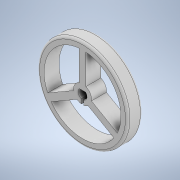
# Autodesk Inventor part: wheel35mmV1
Saved by Autodesk Inventor 2022.2 (Build 262287010, 287A)
## iProperties
Created: 2022-02-20
Part Number: wheel35mmV1
Material: Generic
Document SubType Name: Modeling
Designer: Nakai
Density: 1 g/cm^3
Appearance: Default
Author: Nakai
Autodesk Inventor part; units mm, degrees
ref_plane "YZ Plane" through (0, 0, 0) normal (1, 0, 0) x (0, 1, 0)
ref_plane "XZ Plane" through (0, 0, 0) normal (0, 1, 0) x (-1, 0, 0)
ref_plane "XY Plane" through (0, 0, 0) normal (0, 0, 1) x (1, 0, 0)
sketch "Sketch1" plane through (0, 0, 0) normal (0, 0, 1) x (1, 0, 0)
  circle A0 centre (0, 0) radius 20
  dimension "d0" = 40
  constraints: 1 centre point, 1 coincident
  measures "d0" diameter of A0
extrude "Extrusion1" add sketch "Sketch1" along normal blind 6.6
sketch "Sketch3" plane through (0, 0, 0) normal (0, 0, -1) x (-1, 0, 0)
  circle A0 centre (0, 0) radius 17
  line L0 (0, 17) -> (0, 0)
  line L1 (0, 0) -> (14.7224, -8.5)
  line L2 (0, 0) -> (-14.7224, -8.5)
  line L3 (0, 0) -> (17, 0) construction
  line L4 (1.5, 16.9337) -> (1.5, 0.866)
  line L5 (-1.5, 16.9337) -> (-1.5, 0.866)
  line L6 (-1.5, 0.866) -> (-15.415, -7.1678)
  line L7 (0, -1.7321) -> (-13.915, -9.7659)
  line L8 (1.5, 0.866) -> (15.415, -7.1678)
  line L9 (0, -1.7321) -> (13.915, -9.7659)
  dimension "d6" = 34
  dimension "d7" = 120
  dimension "d8" = 150
  dimension "d9" = 1.5
  dimension "d10" = 1.5
  dimension "d11" = 1.5
  dimension "d12" = 1.5
  dimension "d13" = 1.5
  dimension "d14" = 1.5
  constraints: 20 end point, 6 parallel, 1 coincident, 1 equal length, 1 horizontal, 1 vertical, 11 other
  measures "d7" angle of L1 L0
  measures "d8" angle of L2 L3
  measures "d9" distance between parallel lines of L0 L4
  measures "d10" distance between parallel lines of L0 L5
  measures "d11" distance between parallel lines of L2 L6
  measures "d12" distance between parallel lines of L2 L7
  measures "d13" distance between parallel lines of L1 L8
  measures "d14" distance between parallel lines of L1 L9
extrude "Extrusion3" cut sketch "Sketch3" against normal up to surface (6.6 mm away) contours A0 L8 L4 | L5 L6 A0 | A0 L7 L9
sketch "Sketch5" plane through (0, 0, 6.6) normal (0, 0, 1) x (1, 0, 0)
  circle A0 centre (0, 0) radius 4
  dimension "d20" = 8
  constraints: 1 centre point, 1 coincident
  measures "d20" diameter of A0
extrude "Extrusion5" add sketch "Sketch5" against normal blind 6.6
sketch "Sketch6" plane through (0, 0, 0) normal (0, 0, -1) x (-1, 0, 0)
  circle A0 centre (0, 0) radius 2
  line L0 (0, -2) -> (0, -4)
  arc A1 (-2.4613, -3.1531) -> (2.4613, -3.1531) centre (0, 0) ccw projected
  line L1 (0.5, -1.9365) -> (0.5, -3.9686)
  line L2 (-0.5, -1.9365) -> (-0.5, -3.9686)
  line L3 (-1.3229, 1.5) -> (1.3229, 1.5)
  point P0 (0.0845, 1.5)
  dimension "d23" = 4
  dimension "d24" = 0.5
  dimension "d25" = 0.5
  dimension "d29" = 3.5
  constraints: 8 end point, 8 point on circle, 2 parallel, 1 centre point, 1 coincident, 1 horizontal, 1 point on line, 1 vertical
  measures "d23" diameter of A0
  measures "d24" distance between parallel lines of L0 L1
  measures "d25" distance between parallel lines of L0 L2
  measures "d29" vertical distance of point (0.085, 1.5) L0.start
extrude "Extrusion6" cut sketch "Sketch6" against normal up to surface (6.6 mm away) contours A0 L3 | L1 A1 L0 A0 | L0 A1 L2 A0 picked at (-0.5622, -0.3103)
fillet "Arredondamento1" radius 1 2 edges at (-20, 0, 6.6) (-20, 0, 0)
body "Solid1"
